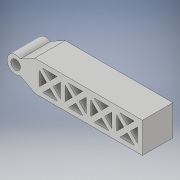
# Autodesk Inventor part: Leg Box
Saved by Autodesk Inventor 2018.2 (Build 222227000, 227)
## iProperties
Created: 2018-02-09
Part Number: Leg Box
Material: Generic
Document SubType Name: Modeling
Designer: MIABo
Density: 1 g/cm^3
Appearance: Default
Mass: 52.5125 g
Surface Area: 166.316 cm^2
Volume: 52.5125 cm^3
Author: MIABo
Autodesk Inventor part; units mm, degrees
ref_plane "YZ Plane" through (0, 0, 0) normal (1, 0, 0) x (0, 1, 0)
sketch "Sketch1" plane through (0, 0, 0) normal (0, 1, 0) x (-1, 0, 0)
  line L0 (7.1935, 4.8681) -> (47.8335, 4.8681)
  line L1 (47.8335, 4.8681) -> (47.8335, -35.7719)
  line L2 (47.8335, -35.7719) -> (7.1935, -35.7719)
  line L3 (7.1935, -35.7719) -> (7.1935, 4.8681)
  point P0 (0, 0)
  point P1 (47.8335, -15.4519)
  dimension "d0" = 40.64
  dimension "d1" = 40.64
  constraints: 8 end point, 1 horizontal, 1 midpoint, 1 parallel, 1 perpendicular, 1 other
  measures "d0" distance of L0.start L0.end
  measures "d1" distance of L0.end L1.end
extrude "Extrusion1" add sketch "Sketch1" along normal blind 6.35
ref_plane "Work Plane1" through (-47.8335, 6.35, 4.8681) normal (-0.7071, -0.7071, 0) x (0, 0, 1)
sketch "Sketch4" plane through (0, 6.35, 0) normal (0, 1, 0) x (1, 0, 0)
  line L0 (-47.8335, -4.8681) -> (-13.5468, -4.8681) projected
  line L1 (-47.8335, 35.7719) -> (-7.1935, 35.7719) projected
  line L2 (-47.8335, -4.8681) -> (-41.4835, -4.8681)
  line L3 (-41.4835, -4.8681) -> (-41.4835, 35.7719)
  line L4 (-41.4835, 35.7719) -> (-47.8335, 35.7719)
  line L5 (-47.8335, 35.7719) -> (-47.8335, -4.8681)
  point P0 (0, 0)
  point P1 (-29.7585, -4.8681)
  dimension "d15" = 6.35
  constraints: 8 end point, 2 parallel, 1 horizontal, 1 perpendicular, 1 point on line
  measures "d15" distance of L4.end L3.end
extrude "Extrusion4" add sketch "Sketch4" along normal blind 34.29
sketch "Sketch5" plane through (0, 6.35, 0) normal (0, 1, 0) x (1, 0, 0)
  line L0 (-7.1935, 35.7719) -> (-13.5435, 35.7719)
  line L1 (-13.5435, 35.7719) -> (-13.5435, -4.8681)
  line L2 (-13.5435, -4.8681) -> (-7.1935, -4.8681)
  line L3 (-7.1935, -4.8681) -> (-7.1935, 35.7719)
  line L4 (-7.1935, -4.8681) -> (-7.1935, 35.7719) projected
  point P0 (0, 0)
  point P1 (-11.6836, 35.7719)
  dimension "d18" = 6.35
  dimension "d19" = 40.64
  constraints: 8 end point, 2 parallel, 1 collinear, 1 horizontal, 1 perpendicular, 1 point on line
  measures "d18" distance of L2.end L1.end
  measures "d19" distance of L1.end L0.end
extrude "Extrusion5" add sketch "Sketch5" along normal blind 34.29
sketch "Sketch6" plane through (-47.8335, 0, 4.8681) normal (0, 0, 1) x (1, 0, 0)
  line L0 (0, 40.64) -> (6.35, 40.64) projected
  line L1 (0, 40.64) -> (40.64, 40.64)
  line L2 (40.64, 40.64) -> (40.64, 34.29)
  line L3 (40.64, 34.29) -> (0, 34.29)
  line L4 (0, 34.29) -> (0, 40.64)
  point P0 (47.8335, 0)
  dimension "d22" = 40.64
  dimension "d23" = 6.35
  constraints: 8 end point, 2 parallel, 1 horizontal, 1 perpendicular
  measures "d22" distance of L2.end L3.end
  measures "d23" distance of L1.end L2.end
extrude "Extrusion6" add sketch "Sketch6" against normal blind 40.64
ref_plane "Work Plane3" through (-7.1935, 6.35, -35.7719) normal (0.7071, -0.7071, 0) x (0, 0, -1)
sketch "Sketch8" plane through (-7.1935, 6.35, -35.7719) normal (0.7071, -0.7071, 0) x (0, 0, -1)
  line L0 (-40.64, -1.3151) -> (-40.64, -7.6651)
  line L1 (-40.64, -4.4901) -> (-40.64, 24.2467) projected
  line L2 (-40.64, -7.6651) -> (0, -7.6651)
  line L3 (0, -33.2269) -> (0, -4.4901) projected
  line L4 (0, -7.6651) -> (0, -1.3151)
  line L5 (0, -1.3151) -> (-40.64, -1.3151)
  dimension "d35" = 6.35
  constraints: 8 end point, 2 vertical, 1 collinear, 1 horizontal, 1 midpoint, 1 perpendicular, 1 point on line
  measures "d35" distance of L2.end L4.end
extrude "Extrusion7" add sketch "Sketch8" against normal blind 48.4886
sketch "Sketch9" plane through (-47.8335, 6.35, 4.8681) normal (-0.7071, -0.7071, 0) x (0, 0, 1)
  line L0 (0, -4.4901) -> (-40.64, -4.4901) projected
  line L1 (0, -4.4901) -> (0, -7.6651)
  line L2 (0, -7.6651) -> (-40.64, -7.6651)
  line L3 (-40.64, -7.6651) -> (-40.64, -1.3151)
  line L4 (-40.64, -1.3151) -> (0, -1.3151)
  line L5 (0, -1.3151) -> (0, -4.4901)
  point P0 (-4.8681, -38.3135)
  dimension "d36" = 3.175
  dimension "d37" = 40.64
  dimension "d38" = 90
  dimension "d39" = 6.35
  dimension "d40" = 90
  dimension "d41" = 40.64
  dimension "d42" = 90
  constraints: 10 end point, 3 perpendicular, 1 vertical
  measures "d36" distance of L0.start L1.end
  measures "d37" distance of L1.end L2.end
  measures "d38" angle of L1 L2
  measures "d39" distance of L2.end L3.end
  measures "d40" angle of L2 L3
  measures "d41" distance of L3.end L4.end
  measures "d42" angle of L3 L4
extrude "Extrusion8" add sketch "Sketch9" against normal blind 48.4886
sketch "Sketch10" plane through (-7.1935, 0, 4.8681) normal (1, 0, 0) x (0, 0, -1)
  line L0 (0, 0) -> (0, 40.64) projected
  line L1 (0, 40.64) -> (40.64, 40.64)
  line L2 (40.64, 40.64) -> (40.64, 0)
  line L3 (40.64, 0) -> (0, 0)
  line L4 (0, 0) -> (0, 40.64)
  point P0 (4.8681, 0)
  constraints: 8 end point, 2 parallel, 1 horizontal, 1 perpendicular
extrude "Extrusion9" cut sketch "Sketch10" against normal blind 3.175
mirror "Mirror1" about plane through (-10.3685, 20.32, -15.4519) normal (1, 0, 0)
sketch "Sketch11" plane through (27.0965, 0, 4.8681) normal (1, 0, 0) x (0, 0, -1)
  line L0 (0, 40.64) -> (40.64, 40.64)
  line L1 (40.64, 40.64) -> (40.64, 0)
  line L2 (40.64, 0) -> (0, 0)
  line L3 (0, 0) -> (0, 40.64)
  point P0 (4.8681, 0)
  dimension "d47" = 40.64
  dimension "d48" = 40.64
  constraints: 8 end point, 2 parallel, 1 horizontal, 1 perpendicular
  measures "d47" distance of L1.end L2.end
  measures "d48" distance of L0.end L1.end
extrude "Extrusion10" cut sketch "Sketch11" against normal blind 3.175
mirror "Mirror2" about plane through (23.9215, 20.32, -15.4519) normal (1, 0, 0)
sketch "Sketch12" plane through (-47.8335, 0, 4.8681) normal (0, 0, 1) x (1, 0, 0)
  circle A0 centre (-25.4, 20.32) radius 6.35
  line L0 (143.51, 40.64) -> (0, 40.64) projected
  line L1 (0, 0) -> (0, 40.64) projected
  line L2 (-19.3329, 30.0069) -> (0, 40.64)
  line L3 (-19.3329, 10.6331) -> (0, 0)
  arc A1 (-19.3329, 30.0069) -> (-19.3329, 10.6331) centre (-25.4, 20.32) ccw
  point P0 (47.8335, 0)
  dimension "d51" = 12.7
  dimension "d52" = 20.32
  dimension "d53" = 25.4
  dimension "d54" = 22.86
  constraints: 4 end point, 2 centre point, 2 point on circle, 1 coincident
  measures "d51" diameter of A0
  measures "d52" distance from line of L0 A0.centre
  measures "d53" distance from line of L1 A0.centre
  measures "d54" diameter of A1
extrude "Extrusion11" add sketch "Sketch12" against normal blind 40.64
body "Solid1"
